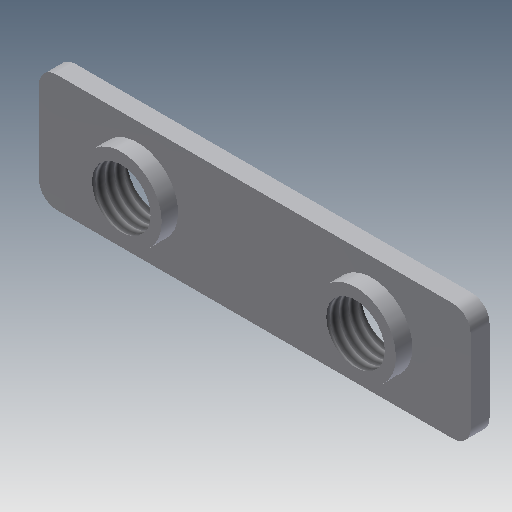
# Autodesk Inventor part: doube t-nut
Saved by Autodesk Inventor 2020.3 (Build 243373000, 373)
## iProperties
Created: 2016-04-11
Part Number: doube t-nut
Material: Generic
Document SubType Name: Modeling
Designer: Ben
Density: 1 g/cm^3
Appearance: Default
Author: Ben
Autodesk Inventor part; units mm, degrees
ref_plane "YZ Plane" through (0, 0, 0) normal (1, 0, 0) x (0, 1, 0)
ref_plane "XZ Plane" through (0, 0, 0) normal (0, 1, 0) x (-1, 0, 0)
ref_plane "XY Plane" through (0, 0, 0) normal (0, 0, 1) x (1, 0, 0)
sketch "Sketch1" plane through (0, 0, 0) normal (0, 0, 1) x (1, 0, 0)
  line L0 (-18.44, 5) -> (18.44, 5)
  line L1 (18.44, 5) -> (18.44, -5)
  line L2 (18.44, -5) -> (-18.44, -5)
  line L3 (-18.44, -5) -> (-18.44, 5)
  line L4 (0, 5) -> (0, -5) construction
  line L5 (-18.44, 0) -> (18.44, 0) construction
  circle A0 centre (-10, 0) radius 2.5
  circle A1 centre (10, 0) radius 2.5
  point P0 (0, 0)
  dimension "d0" = 10
  dimension "d1" = 36.88
  dimension "d2" = 5
  dimension "d3" = 20
  constraints: 12 end point, 6 midpoint, 2 centre point, 2 parallel, 1 horizontal, 1 perpendicular, 1 point on line, 1 symmetric about line, 1 other
  measures "d0" distance of L0.end L1.end
  measures "d1" distance of L0.start L0.end
  measures "d2" diameter of A0
  measures "d3" distance of A1.centre A0.centre
extrude "Extrusion1" add sketch "Sketch1" along normal blind 1.6
sketch "Sketch2" plane through (0, 0, 1.6) normal (0, 0, 1) x (1, 0, 0)
  circle A0 centre (10, 0) radius 2.5 projected
  circle A1 centre (-10, 0) radius 2.5 projected
  circle A2 centre (-10, 0) radius 3.45
  circle A3 centre (10, 0) radius 3.45
  point P0 (0, 0)
  dimension "d6" = 6.9
  dimension "d7" = 6.9
  constraints: 2 centre point, 2 coincident
  measures "d6" diameter of A2
  measures "d7" diameter of A3
extrude "Extrusion2" add sketch "Sketch2" along normal blind 1.4
thread "Thread1" size "M5x0.8" class "6H" standard "ANSI Metric M Profile" full length
thread "Thread2" size "M5x0.8" class "6H" standard "ANSI Metric M Profile" full length
fillet "Fillet1" radius 1.51 4 edges at (18.44, 5, 0.8) (18.44, -5, 0.8) (-18.44, -5, 0.8) (-18.44, 5, 0.8)
body "Solid1"
